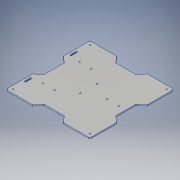
# Autodesk Inventor part: Heated Bed Plate
Saved by Autodesk Inventor 2019.4 (Build 234330000, 330)
## iProperties
Created: 2018-08-19
Part Number: Heated Bed Plate
Material: Aluminum 6061
Document SubType Name: Modeling
Designer: Richard
Density: 2.7 g/cm^3
Appearance: Aluminum - Flat
Author: Richard
Autodesk Inventor part; units mm, degrees
ref_plane "YZ Plane" through (0, 0, 0) normal (1, 0, 0) x (0, 1, 0)
ref_plane "XZ Plane" through (0, 0, 0) normal (0, 1, 0) x (-1, 0, 0)
ref_plane "XY Plane" through (0, 0, 0) normal (0, 0, 1) x (1, 0, 0)
sketch "Sketch1" plane through (0, 0, 0) normal (0, 1, 0) x (-1, 0, 0)
  line L0 (114.5, 114.5) -> (-114.5, 114.5)
  line L1 (-114.5, 114.5) -> (-114.5, -114.5)
  line L2 (-114.5, -114.5) -> (114.5, -114.5)
  line L3 (114.5, -114.5) -> (114.5, 114.5)
  line L4 (114.5, 114.5) -> (-114.5, -114.5) construction
  line L5 (-114.5, 114.5) -> (114.5, -114.5) construction
  point P0 (0, 0)
  dimension "d0" = 229
  constraints: 12 end point, 2 midpoint, 2 parallel, 2 perpendicular, 1 horizontal
  measures "d0" distance of L2.end L0.start
extrude "Extrusion1" add sketch "Sketch1" along normal mid plane 3.175
sketch "Sketch2" plane through (0, 1.5875, 0) normal (0, 1, 0) x (1, 0, 0)
  line L0 (-114.5, -114.5) -> (114.5, -114.5) construction
  line L1 (114.5, -114.5) -> (114.5, 114.5) construction
  line L2 (114.5, 114.5) -> (-114.5, 114.5) construction
  line L3 (-114.5, 114.5) -> (-114.5, -114.5) construction
  line L4 (-41.7647, 114.5) -> (-27.5, 97.5)
  line L5 (-27.5, 97.5) -> (27.5, 97.5)
  line L6 (27.5, 97.5) -> (41.7647, 114.5)
  line L7 (41.7647, 114.5) -> (-41.7647, 114.5)
  line L8 (-97.5, -27.5) -> (-97.5, 27.5)
  line L9 (-114.5, -41.7647) -> (-97.5, -27.5)
  line L10 (-114.5, 41.7647) -> (-114.5, -41.7647)
  line L11 (-97.5, 27.5) -> (-114.5, 41.7647)
  line L12 (27.5, -97.5) -> (-27.5, -97.5)
  line L13 (41.7647, -114.5) -> (27.5, -97.5)
  line L14 (-41.7647, -114.5) -> (41.7647, -114.5)
  line L15 (-27.5, -97.5) -> (-41.7647, -114.5)
  line L16 (97.5, 27.5) -> (97.5, -27.5)
  line L17 (114.5, 41.7647) -> (97.5, 27.5)
  line L18 (114.5, -41.7647) -> (114.5, 41.7647)
  line L19 (97.5, -27.5) -> (114.5, -41.7647)
  line L20 (-106.5, 69.5) -> (-106.5, 54.5) construction
  line L21 (-108.5, 69.5) -> (-108.5, 54.5)
  line L22 (-104.5, 54.5) -> (-104.5, 69.5)
  arc A0 (-104.5, 69.5) -> (-108.5, 69.5) centre (-106.5, 69.5) ccw
  arc A1 (-108.5, 54.5) -> (-104.5, 54.5) centre (-106.5, 54.5) ccw
  line L23 (0, 0) -> (-31.1886, 0)
  line L24 (-108.5, -69.5) -> (-108.5, -54.5)
  line L25 (-104.5, -54.5) -> (-104.5, -69.5)
  arc A2 (-108.5, -69.5) -> (-104.5, -69.5) centre (-106.5, -69.5) ccw
  arc A3 (-104.5, -54.5) -> (-108.5, -54.5) centre (-106.5, -54.5) ccw
  point P0 (0, 114.5)
  point P1 (-114.5, 0)
  point P2 (0, -114.5)
  point P3 (114.5, 0)
  point P4 (-106.5, 62)
  dimension "d5" = 55
  dimension "d8" = 360
  dimension "d10" = 195
  dimension "d32" = 4
  dimension "d33" = 15
  dimension "d34" = 52.5
  dimension "d35" = 6
  dimension "d36" = 50
  constraints: 46 end point, 8 point on circle, 6 symmetric about line, 4 centre point, 4 tangent, 2 horizontal, 2 midpoint, 1 collinear, 1 equal length, 1 parallel, 1 vertical, 1 vertical alignment, 39 other
  measures "d5" distance of L4.end L5.end
  measures "d10" distance between parallel lines of L12 L5
  measures "d32" distance between parallel lines of L22 L21
  measures "d33" distance of L20.start L20.end
  measures "d34" distance edge to line of A1 L23
  measures "d35" distance between parallel lines of L3 L21
  measures "d36" angle of L5 L6
extrude "Extrusion2" cut sketch "Sketch2" against normal blind 3.175
chamfer "Chamfer1" distance 4 angle 45 4 edges at (-114.5, 0, 114.5) (-114.5, 0, -114.5) (114.5, 0, -114.5) (114.5, 0, 114.5)
sketch "Sketch3" plane through (0, 1.5875, 0) normal (0, 1, 0) x (1, 0, 0)
  line L0 (-104.5, -104.5) -> (104.5, -104.5) construction
  line L1 (104.5, -104.5) -> (104.5, 104.5) construction
  line L2 (104.5, 104.5) -> (-104.5, 104.5) construction
  line L3 (-104.5, 104.5) -> (-104.5, -104.5) construction
  line L4 (-104.5, -104.5) -> (104.5, 104.5) construction
  line L5 (104.5, -104.5) -> (-104.5, 104.5) construction
  line L6 (-78.5, 50) -> (-46.5, 50) construction
  line L7 (-78.5, -50) -> (-46.5, -50) construction
  line L8 (46.5, 0) -> (78.5, 0) construction
  point P0 (0, 0)
  point P1 (0, 0)
  dimension "d16" = 209
  dimension "d17" = 209
  dimension "d18" = 32
  dimension "d20" = 46.5
  dimension "d21" = 46.5
  dimension "d22" = 100
  dimension "d23" = 50
  dimension "d24" = 93
  constraints: 18 end point, 10 coincident, 4 horizontal, 4 parallel, 3 midpoint, 1 perpendicular, 1 point on line, 1 vertical alignment
  measures "d16" distance of L2.end L1.end
  measures "d17" distance of L1.end L0.end
  measures "d18" distance of L6.start L6.end
  measures "d20" horizontal distance of point (0, 0) L6.end
  measures "d21" distance of L8.start point (0, 0)
  measures "d22" distance between parallel lines of L7 L6
  measures "d23" distance from line of point (0, 0) L6
  measures "d24" horizontal distance of L8.start L6.end
hole "Hole1" at (-104.5, 1.5875, -104.5) at (104.5, 1.5875, -104.5) at (104.5, 1.5875, 104.5) at (-104.5, 1.5875, 104.5) at (-78.5, 1.5875, -50) at (-46.5, 1.5875, -50) at (46.5, 1.5875, 0) at (78.5, 1.5875, 0) at (-46.5, 1.5875, 50) at (-78.5, 1.5875, 50) direction (0, -1, 0) diameter 3.2 end through all start extended yes
fillet "Fillet1" radius 1.27 16 edges at (-114.5, 0, -41.7647) (-97.5, 0, -27.5) (-97.5, 0, 27.5) (-114.5, 0, 41.7647) (-27.5, 0, 97.5) (27.5, 0, 97.5) (41.7647, 0, 114.5) (-41.7647, 0, 114.5) (114.5, 0, -41.7647) (97.5, 0, -27.5) (97.5, 0, 27.5) (114.5, 0, 41.7647) (-41.7647, 0, -114.5) (-27.5, 0, -97.5) (27.5, 0, -97.5) (41.7647, 0, -114.5)
sketch "Sketch4" plane through (0, 1.5875, 0) normal (0, 1, 0) x (1, 0, 0)
  line L0 (-3.5, 22.5) -> (-3.5, -22.5)
  line L1 (-114.5, 110.5) -> (-114.5, 42.3569) projected
  point P0 (0, 0)
  point P1 (-3.5, 0)
  dimension "d38" = 45
  dimension "d39" = 111
  constraints: 2 coincident, 2 end point, 1 horizontal alignment, 1 midpoint, 1 vertical
  measures "d38" distance of L0.start L0.end
  measures "d39" distance between parallel lines of L1 L0
hole "Hole2" at (-3.5, 1.5875, -22.5) at (-3.5, 1.5875, 22.5) direction (0, -1, 0) diameter 3.4036 depth 6.4 clearance for "Flat Head Machine Screw" size "M3" standard "Ansi Metric M Profile"
equation "\"d21\" = d20"
body "Solid1"
